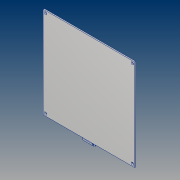
# Autodesk Inventor part: Heated bed
Saved by Autodesk Inventor 2019 (Build 230136000, 136)
## iProperties
Created: 2018-11-26
Part Number: Heated bed
Material: Aluminum 6061
Document SubType Name: Modeling
Designer: LillaHunden
Density: 2.7 g/cm^3
Appearance: Aluminum - Flat
Author: LillaHunden
Autodesk Inventor part; units mm, degrees
ref_plane "YZ Plane" through (0, 0, 0) normal (1, 0, 0) x (0, 1, 0)
ref_plane "XZ Plane" through (0, 0, 0) normal (0, 1, 0) x (-1, 0, 0)
ref_plane "XY Plane" through (0, 0, 0) normal (0, 0, 1) x (1, 0, 0)
sketch "Sketch1" plane through (0, 0, 0) normal (0, 0, 1) x (1, 0, 0)
  line L0 (-110, -110) -> (110, -110)
  line L1 (110, -110) -> (110, 110)
  line L2 (110, 110) -> (-110, 110)
  line L3 (-110, 110) -> (-110, -110)
  line L4 (-110, -110) -> (110, 110) construction
  line L5 (110, -110) -> (-110, 110) construction
  point P0 (0, 0)
  dimension "d0" = 220
  dimension "d1" = 220
  constraints: 12 end point, 2 midpoint, 2 parallel, 1 horizontal, 1 perpendicular
  measures "d0" distance of L2.end L1.end
  measures "d1" distance of L1.end L0.end
extrude "Extrusion1" add sketch "Sketch1" along normal blind 3
sketch "Sketch2" plane through (0, 0, 3) normal (0, 0, 1) x (1, 0, 0)
  line L0 (0, 0) -> (0, 31.036)
  line L1 (0, 0) -> (15.0174, 0)
  point P0 (-104.5, 104.5)
  point P1 (104.5, 104.5)
  point P2 (104.5, -104.5)
  point P3 (-104.5, -104.5)
  dimension "d4" = 209
  dimension "d5" = 209
  constraints: 4 end point, 2 horizontal alignment, 2 symmetric about line, 2 vertical alignment, 1 horizontal, 1 vertical
  measures "d4" distance of point (-104.5, -104.5) point (-104.5, 104.5)
  measures "d5" distance of point (-104.5, 104.5) point (104.5, 104.5)
hole "Hole1" at (-104.5, 104.5, 3) at (104.5, 104.5, 3) at (104.5, -104.5, 3) at (-104.5, -104.5, 3) direction (0, 0, -1) diameter 3.4 depth 7.25 tip angle 118 countersink diameter 6.3 countersink angle 90 clearance for "Countersunk Flat Head Screw ISO 2009/7046" size "M3" standard "ISO"
ref_plane "Work Plane1" through (-15, -110, 0) normal (-1, 0, 0) x (0, 0, 1)
sketch "Sketch3" plane through (-15, -110, 0) normal (-1, 0, 0) x (0, 0, 1)
  line L0 (4.5, 0) -> (-3.7, 0)
  line L1 (-3.7, 0) -> (-3.7, -3)
  line L2 (-3.7, -3) -> (4.5, -3)
  line L3 (4.5, -3) -> (4.5, 0)
  line L4 (3, 8.65) -> (3, 2.35) construction
  line L5 (3, 217.65) -> (3, 211.35) construction
  line L6 (3, 217.65) -> (3, 211.35) construction
  line L7 (3, 8.65) -> (3, 2.35) construction
  line L8 (3, 0) -> (3, 220) construction
  line L9 (3, 220) -> (3, 0) construction
  line L10 (0, 3.8) -> (0, 7.2) construction
  line L11 (0, 212.8) -> (0, 216.2) construction
  line L12 (0, 212.8) -> (0, 216.2) construction
  line L13 (0, 3.8) -> (0, 7.2) construction
  line L14 (0, 220) -> (0, 0) construction
  line L15 (0, 0) -> (0, 220) construction
  point P0 (0, 110)
  dimension "d14" = 3
  dimension "d15" = 8.2
  dimension "d16" = 1.5
  constraints: 8 end point, 2 parallel, 1 horizontal, 1 horizontal alignment, 1 perpendicular
  measures "d14" distance of L2.end L0.start
  measures "d15" distance of L1.end L2.end
  measures "d16" distance between parallel lines of L8 L3
extrude "Extrusion2" add sketch "Sketch3" against normal blind 24
sketch "Sketch5" plane through (9, -110, 0) normal (1, 0, 0) x (0, 0, -1)
  line L0 (3.7, -3) -> (-4.5, -3) projected
  line L1 (3.1753, -3) -> (3.1753, -9.1)
  line L2 (3.1753, -9.1) -> (3.5377, -9.2206)
  line L3 (3.5377, -9.2206) -> (3.7, -9.2206)
  line L4 (3.7, -9.2206) -> (3.8268, -8.836)
  line L5 (3.8268, -8.836) -> (3.7, -8.836)
  line L6 (3.7, -8.836) -> (3.7, -3)
  line L7 (-4.5, -3) -> (3.7, -3) projected
  line L8 (3.7, -3) -> (3.1753, -3)
  point P0 (0, 110)
  dimension "d30" = 6.1
  constraints: 14 end point, 1 collinear, 1 parallel, 1 perpendicular, 1 point on line, 1 vertical
  measures "d30" distance of L1.start L1.end
extrude "Extrusion4" add sketch "Sketch5" against normal up to surface (24 mm away)
sketch "Sketch4" plane through (-15, -110, 0) normal (0, 1, 0) x (1, 0, 0)
  line L0 (1.3075, 0.9305) -> (2.4075, 0.9305)
  line L1 (2.4075, 0.9305) -> (2.4075, -0.1695)
  line L2 (2.4075, -0.1695) -> (1.3075, -0.1695)
  line L3 (1.3075, -0.1695) -> (1.3075, 0.9305)
  line L4 (5.4075, 0.9305) -> (6.5075, 0.9305)
  line L5 (6.5075, 0.9305) -> (6.5075, -0.1695)
  line L6 (6.5075, -0.1695) -> (5.4075, -0.1695)
  line L7 (5.4075, -0.1695) -> (5.4075, 0.9305)
  line L8 (9.5075, 0.9305) -> (10.6075, 0.9305)
  line L9 (10.6075, 0.9305) -> (10.6075, -0.1695)
  line L10 (10.6075, -0.1695) -> (9.5075, -0.1695)
  line L11 (9.5075, -0.1695) -> (9.5075, 0.9305)
  line L12 (13.6075, 0.9305) -> (14.7075, 0.9305)
  line L13 (14.7075, 0.9305) -> (14.7075, -0.1695)
  line L14 (14.7075, -0.1695) -> (13.6075, -0.1695)
  line L15 (13.6075, -0.1695) -> (13.6075, 0.9305)
  line L16 (17.7075, 0.9305) -> (18.8075, 0.9305)
  line L17 (18.8075, 0.9305) -> (18.8075, -0.1695)
  line L18 (18.8075, -0.1695) -> (17.7075, -0.1695)
  line L19 (17.7075, -0.1695) -> (17.7075, 0.9305)
  line L20 (21.8075, 0.9305) -> (22.9075, 0.9305)
  line L21 (22.9075, 0.9305) -> (22.9075, -0.1695)
  line L22 (22.9075, -0.1695) -> (21.8075, -0.1695)
  line L23 (21.8075, -0.1695) -> (21.8075, 0.9305)
  point P0 (15, 0)
  dimension "d19" = 1.1
  dimension "d20" = 1.1
  dimension "d23" = 4.1
  constraints: 48 end point, 2 horizontal, 2 parallel, 1 collinear, 1 perpendicular, 39 other
  measures "d19" distance of L0.start L0.end
  measures "d20" distance of L0.end L1.end
  measures "d23" distance of L0.start L4.start
extrude "Extrusion3" add sketch "Sketch4" along normal blind 8 and the other way blind 7.75
equation "\"d20\" = d19"
body "Solid1"
